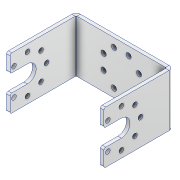
# Autodesk Inventor part: bottom
Saved by Autodesk Inventor 2020 (Build 240168000, 168)
## iProperties
Created: 2020-11-05
Part Number: bottom
Material: 알루미늄 6061
Document SubType Name: Sheet Metal
Designer: 이호석
Mass: 18.9238 g
Surface Area: 81.3593 cm^2
Volume: 7.00882 cm^3
Density: 2.7 g/cm^3
Sheet Metal Rule: 기본값_mm
Appearance: 알루미늄 - 평지
Author: 이호석
Autodesk Inventor part; units mm, degrees
ref_plane "YZ Plane" through (0, 0, 0) normal (1, 0, 0) x (0, 1, 0)
ref_plane "XZ Plane" through (0, 0, 0) normal (0, 1, 0) x (-1, 0, 0)
ref_plane "XY Plane" through (0, 0, 0) normal (0, 0, 1) x (1, 0, 0)
sketch "스케치1" plane through (0, 0, 0) normal (0, 0, 1) x (1, 0, 0)
  line L0 (28, -15) -> (-28, -15)
  line L1 (-28, -15) -> (-28, 15)
  line L2 (-28, 15) -> (28, 15)
  line L3 (28, 15) -> (28, -15)
  line L4 (28, -15) -> (-28, 15) construction
  line L5 (-28, -15) -> (28, 15) construction
  point P0 (0, 0)
  dimension "d0" = 56
  dimension "d1" = 30
  measures "d0" distance of L1.end L2.end
  measures "d1" distance of L0.end L1.end
extrude "판1" add sketch "스케치1" along normal blind 2
sketch "스케치2" plane through (-28, -15, 2.5) normal (1, 0, 0) x (0, 1, 0)
  line L0 (30, -0.5) -> (0, -0.5)
  line L1 (0, -0.5) -> (0, 37.5)
  line L2 (0, 37.5) -> (30, 37.5)
  line L3 (30, 37.5) -> (30, -0.5)
  constraints: 8 end point
edge flange "플랜지1" height 40 angle 90 thickness 2 bend radius 0.5 thickness toward (1, 0, 0) relief tear relief width 2 relief depth 1 edges at (-28, 0, 2) wall of the first edge with corners at (-28, 15, 2) (-28, -15, 2) (-28, -15, 40) (-28, 15, 40)
bend "절곡부1"
corner "구석1"
sketch "스케치3" plane through (28, 15, 2.5) normal (-1, 0, 0) x (0, -1, 0)
  line L0 (30, -0.5) -> (0, -0.5)
  line L1 (0, -0.5) -> (0, 37.5)
  line L2 (0, 37.5) -> (30, 37.5)
  line L3 (30, 37.5) -> (30, -0.5)
  constraints: 8 end point
edge flange "플랜지2" height 40 angle 90 thickness 2 bend radius 0.5 thickness toward (-1, 0, 0) relief tear relief width 2 relief depth 1 edges at (28, 0, 2) wall of the first edge with corners at (28, -15, 2) (28, 15, 2) (28, 15, 40) (28, -15, 40)
bend "절곡부2"
corner "구석2"
sketch "스케치4" plane through (0, 0, 2) normal (0, 0, 1) x (1, 0, 0)
  circle A0 centre (0, 0) radius 11
  line L0 (0, 0) -> (10.1627, 4.2095)
  line L1 (0, 0) -> (11, 0) construction
  circle A1 centre (10.1627, 4.2095) radius 1.5
  circle A2 centre (4.2095, 10.1627) radius 1.5
  circle A3 centre (-4.2095, 10.1627) radius 1.5
  circle A4 centre (-10.1627, 4.2095) radius 1.5
  circle A5 centre (-10.1627, -4.2095) radius 1.5
  circle A6 centre (-4.2095, -10.1627) radius 1.5
  circle A7 centre (4.2095, -10.1627) radius 1.5
  circle A8 centre (10.1627, -4.2095) radius 1.5
  dimension "d23" = 22
  dimension "d25" = 11
  dimension "d26" = 22.5
  dimension "d27" = 3
  dimension "d30" = 360
  constraints: 9 centre point, 4 end point, 2 coincident, 1 equal length, 1 horizontal, 17 other
  measures "d23" diameter of A0
  measures "d25" distance of L0.start L0.end
  measures "d26" angle of L1 L0
  measures "d27" diameter of A1
extrude "돌출1" cut sketch "스케치4" against normal through all contours A1 L0 A0 | A0 A1 | A8 A0 | A0 A8 | L0 A1 A0 | A7 A0 | A0 A7 | A2 A0 | A0 A2 | A6 A0 | A0 A6 | A3 A0 | A0 A3 | A5 A0 | A0 A5 | A4 A0 | A0 A4
sketch "스케치5" plane through (28, -15, 40) normal (1, 0, 0) x (0, 0, -1)
  line L0 (37.5, 0) -> (0, 0) projected
  line L1 (0, 0) -> (0, 30) projected
  line L2 (15, 15) -> (10, 15)
  arc A0 (10, 10) -> (10, 20) centre (10, 15) ccw
  line L3 (10, 20) -> (0, 20)
  line L4 (10, 10) -> (0, 10)
  line L5 (10, 15) -> (10, 4)
  circle A1 centre (10, 4) radius 1.35
  circle A2 centre (17.7782, 7.2218) radius 1.35
  circle A3 centre (21, 15) radius 1.35
  circle A4 centre (17.7782, 22.7782) radius 1.35
  circle A5 centre (10, 26) radius 1.35
  circle A6 centre (2.2218, 22.7782) radius 1.35
  circle A7 centre (-1, 15) radius 1.35
  circle A8 centre (2.2218, 7.2218) radius 1.35
  point P0 (40, 15)
  point P1 (0, 14.0931)
  point P2 (0, 15.9069)
  dimension "d35" = 5
  dimension "d36" = 11
  dimension "d37" = 2.7
  dimension "d40" = 360
  constraints: 9 centre point, 8 end point, 3 point on circle, 3 point on line, 2 coincident, 1 parallel, 1 perpendicular, 1 tangent, 1 vertical, 17 other
  measures "d35" distance of L2.start L2.end
  measures "d36" distance of L5.start L5.end
  measures "d37" diameter of A1
extrude "돌출2" cut sketch "스케치5" against normal through all
fillet "모서리 라운드1" radius 1 8 edges at (27, -5, 40) (27, 15, 40) (-27, 15, 40) (-27, -5, 40) (-27, 5, 40) (27, 5, 40) (27, -15, 40) (-27, -15, 40)
equation "\"d3\" = BendReliefWidth"
equation "\"d4\" = BendReliefDepth"
equation "\"d5\" = MinimumRemnant"
equation "\"d6\" = TransitionRadius"
equation "\"d10\" = CornerReliefSize"
equation "\"d13\" = BendReliefWidth"
equation "\"d14\" = BendReliefDepth"
equation "\"d15\" = MinimumRemnant"
equation "\"d16\" = TransitionRadius"
equation "\"d20\" = CornerReliefSize"
equation "\"TransitionRadius\" = BendRadius"
equation "\"BendReliefWidth\" = 2"
equation "\"BendReliefDepth\" = 1"
equation "\"MinimumRemnant\" = 4"
equation "\"CornerReliefSize\" = 8"
equation "\"BendRadius\" = 2"
